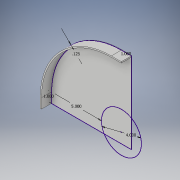
# Autodesk Inventor part: shooter shell
Saved by Autodesk Inventor 2019 (Build 230136000, 136)
## iProperties
Created: 2020-09-22
Part Number: shooter shell
Material: Generic
Document SubType Name: Modeling
Designer: Delta
Density: 1 g/cm^3
Appearance: Default
Author: Delta
Autodesk Inventor part; units mm, degrees
ref_plane "YZ Plane" through (0, 0, 0) normal (1, 0, 0) x (0, 1, 0)
ref_plane "XZ Plane" through (0, 0, 0) normal (0, 1, 0) x (-1, 0, 0)
ref_plane "XY Plane" through (0, 0, 0) normal (0, 0, 1) x (1, 0, 0)
sketch "Sketch1" plane through (0, 0, 0) normal (0, 0, 1) x (1, 0, 0)
  circle A0 centre (0, 0) radius 50.8
  arc A1 (0, 177.8) -> (-177.8, 0) centre (0, 0) ccw
  line L0 (0, 177.8) -> (25.4, 177.8)
  line L1 (-177.8, 0) -> (-177.8, -25.4)
  line L2 (-180.975, -25.4) -> (-180.975, 0)
  arc A2 (0, 180.975) -> (-180.975, 0) centre (0, 0) ccw
  line L3 (0, 180.975) -> (25.4, 180.975)
  line L4 (25.4, 180.975) -> (25.4, 177.8)
  line L5 (-180.975, -25.4) -> (-177.8, -25.4)
  line L6 (-177.8, -25.4) -> (25.4, -25.4)
  line L7 (25.4, -25.4) -> (25.4, 177.8)
  dimension "d0" = 101.6
  dimension "d1" = 127
  dimension "d2" = 25.4
  dimension "d3" = 25.4
  dimension "d4" = 3.175
  constraints: 16 end point, 4 point on circle, 3 centre point, 2 horizontal, 2 perpendicular, 2 tangent, 2 vertical, 1 coincident, 2 other
  measures "d0" diameter of A0
  measures "d1" radial gap between concentric circles of A0 A1
  measures "d2" distance of L0.start L0.end
  measures "d3" distance of L1.start L1.end
  measures "d4" radial gap between concentric circles of A1 A2
extrude "Extrusion1" add sketch "Sketch1" along normal blind 25.4 contours L0 A1 L1 L5 L2 A2 L3 L4
extrude "Extrusion2" add sketch "Sketch1" against normal blind 1.524 contours L7 L6 A0 | A0 L6 L1 A1 L0 L7 | L0 A1 L1 L5 L2 A2 L3 L4 picked at (-13.0459, 17.498)
body "Solid1"
